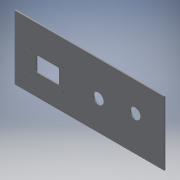
# Autodesk Inventor part: LFEV2017_TSI_003
Saved by Autodesk Inventor 2017 (Build 210142000, 142)
## iProperties
Created: 2017-04-03
Part Number: LFEV2017_TSI_003
Material: Generic
Document SubType Name: Modeling
Designer: hoeflinc
Density: 1 g/cm^3
Appearance: Default
Material_size: Steel   Thickness: .125"
Quantity: 1
Author: hoeflinc
Autodesk Inventor part; units mm, degrees
ref_plane "YZ Plane" through (0, 0, 0) normal (1, 0, 0) x (0, 1, 0)
ref_plane "XZ Plane" through (0, 0, 0) normal (0, 1, 0) x (-1, 0, 0)
ref_plane "XY Plane" through (0, 0, 0) normal (0, 0, 1) x (1, 0, 0)
sketch "Sketch1" plane through (0, 0, 0) normal (0, 0, 1) x (1, 0, 0)
  line L0 (0, 0) -> (355.6, 0)
  line L1 (355.6, 0) -> (355.6, 152.4)
  line L2 (355.6, 152.4) -> (0, 152.4)
  line L3 (0, 152.4) -> (0, 0)
  dimension "d0" = 152.4
  dimension "d1" = 355.6
  constraints: 8 end point, 2 parallel, 1 horizontal, 1 perpendicular
  measures "d0" distance of L2.end L0.start
  measures "d1" distance of L0.start L0.end
extrude "Extrusion1" add sketch "Sketch1" along normal blind 3.175
sketch "Sketch2" plane through (0, 0, 3.175) normal (0, 0, 1) x (1, 0, 0)
  line L0 (50.8, 50.8) -> (105.918, 50.8)
  line L1 (105.918, 50.8) -> (105.918, 86.36)
  line L2 (105.918, 86.36) -> (50.8, 86.36)
  line L3 (50.8, 86.36) -> (50.8, 50.8)
  line L4 (0, 152.4) -> (0, 0) projected
  line L5 (0, 0) -> (355.6, 0) projected
  dimension "d4" = 55.118
  dimension "d5" = 35.56
  dimension "d6" = 50.8
  dimension "d7" = 50.8
  constraints: 8 end point, 2 parallel, 1 horizontal, 1 perpendicular
  measures "d4" distance of L0.start L0.end
  measures "d5" distance of L2.end L0.start
  measures "d6" distance between parallel lines of L4 L3
  measures "d7" distance between parallel lines of L5 L0
extrude "Extrusion2" cut sketch "Sketch2" against normal blind 3.175
sketch "Sketch3" plane through (0, 0, 3.175) normal (0, 0, 1) x (1, 0, 0)
  circle A0 centre (199.136, 69.85) radius 12.7
  circle A1 centre (286.5628, 82.804) radius 12.7
  line L0 (0, 0) -> (355.6, 0) projected
  line L1 (0, 152.4) -> (0, 0) projected
  line L2 (355.6, 0) -> (355.6, 152.4) projected
  dimension "d10" = 25.4
  dimension "d11" = 25.4
  dimension "d12" = 69.85
  dimension "d13" = 82.804
  dimension "d14" = 199.136
  dimension "d15" = 69.0372
  constraints: 2 centre point
  measures "d10" diameter of A1
  measures "d11" diameter of A0
  measures "d12" distance from line of L0 A0.centre
  measures "d13" distance from line of L0 A1.centre
  measures "d14" distance from line of A0.centre L1
  measures "d15" distance from line of A1.centre L2
extrude "Extrusion3" cut sketch "Sketch3" against normal blind 3.175
sketch "Sketch4" plane through (0, 0, 3.175) normal (0, 0, 1) x (1, 0, 0)
  line L0 (0, 0) -> (355.6, 0) projected
  line L1 (0, 152.4) -> (0, 0) projected
  point P0 (40.64, 41.91)
  point P1 (116.84, 41.91)
  point P2 (116.84, 92.71)
  point P3 (40.64, 92.71)
  dimension "d18" = 41.91
  dimension "d19" = 41.91
  dimension "d20" = 92.71
  dimension "d21" = 92.71
  dimension "d22" = 40.64
  dimension "d23" = 116.84
  dimension "d24" = 40.64
  dimension "d25" = 116.84
  measures "d18" distance from line of point (40.64, 41.91) L0
  measures "d19" distance from line of point (116.84, 41.91) L0
  measures "d20" distance from line of point (40.64, 92.71) L0
  measures "d21" distance from line of point (116.84, 92.71) L0
  measures "d22" distance from line of L1 point (40.64, 92.71)
  measures "d23" distance from line of L1 point (116.84, 92.71)
  measures "d24" distance from line of L1 point (40.64, 41.91)
  measures "d25" distance from line of L1 point (116.84, 41.91)
hole "Hole1" at (40.64, 41.91, 3.175) at (116.84, 41.91, 3.175) at (116.84, 92.71, 3.175) at (40.64, 92.71, 3.175) direction (0, 0, -1) diameter 3.302 end through all thread size "8-32 UNC" class "2B" standard "ANSI Unified Screw Threads"
fillet "Fillet1" radius 3.175 4 edges at (50.8, 50.8, 1.5875) (105.918, 86.36, 1.5875) (105.918, 50.8, 1.5875) (50.8, 86.36, 1.5875)
equation "\"d19\" = d18"
equation "\"d21\" = d20"
equation "\"d24\" = d22"
equation "\"d25\" = d23"
body "Solid1"
